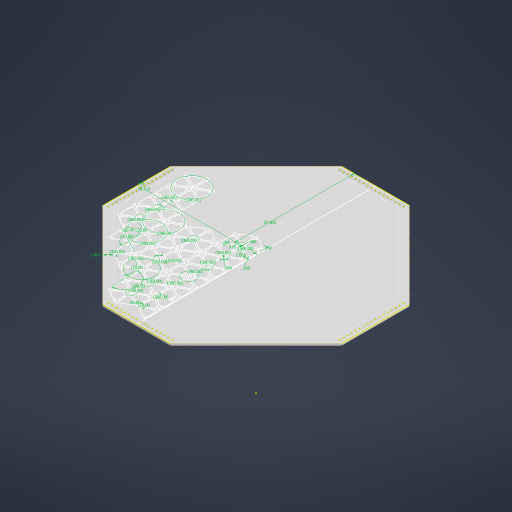
# Autodesk Inventor part: Belly Pan
Saved by Autodesk Inventor 2024.3 (Build 283343000, 343)
## iProperties
Created: 2024-11-27
Part Number: Belly Pan
Material: Generic
Document SubType Name: Modeling
Designer: kaito
Density: 1 g/cm^3
Appearance: Default
Author: kaito
Autodesk Inventor part; units mm, degrees
(part 1 of 2)
ref_plane "YZ Plane" through (0, 0, 0) normal (1, 0, 0) x (0, 1, 0)
ref_plane "XZ Plane" through (0, 0, 0) normal (0, 1, 0) x (-1, 0, 0)
ref_plane "XY Plane" through (0, 0, 0) normal (0, 0, 1) x (1, 0, 0)
sketch "Sketch1" plane through (0, 0, 0) normal (0, 1, 0) x (-1, 0, 0)
  line L0 (0, 0) -> (762, 0) construction
  line L1 (762, 0) -> (762, -762)
  line L2 (762, -762) -> (0, -762)
  line L3 (762, -273.05) -> (736.6, -273.05) construction
  line L4 (736.6, -273.05) -> (736.6, -488.95) construction
  line L5 (736.6, -488.95) -> (762, -488.95) construction
  line L6 (762, -488.95) -> (762, -273.05) construction
  line L7 (488.95, 0) -> (273.05, 0)
  line L8 (273.05, 0) -> (273.05, -25.4) construction
  line L9 (273.05, -25.4) -> (488.95, -25.4) construction
  line L10 (488.95, -25.4) -> (488.95, 0) construction
  line L11 (488.95, -762) -> (273.05, -762) construction
  line L12 (273.05, -762) -> (273.05, -736.6) construction
  line L13 (273.05, -736.6) -> (488.95, -736.6) construction
  line L14 (488.95, -736.6) -> (488.95, -762) construction
  line L15 (0, 0) -> (0, -762)
  line L16 (0, -273.05) -> (25.4, -273.05) construction
  line L17 (25.4, -273.05) -> (25.4, -488.95) construction
  line L18 (25.4, -488.95) -> (0, -488.95) construction
  line L19 (0, -488.95) -> (0, -273.05) construction
  line L20 (273.05, 0) -> (0, -273.05)
  line L21 (488.95, 0) -> (762, -273.05)
  line L22 (762, -488.95) -> (488.95, -762)
  line L23 (0, -488.95) -> (273.05, -762)
  circle A0 centre (482.6, -12.7) radius 2.4892
  circle A1 centre (469.9, -12.7) radius 2.4892
  circle A2 centre (457.2, -12.7) radius 2.4892
  circle A3 centre (444.5, -12.7) radius 2.4892
  circle A4 centre (431.8, -12.7) radius 2.4892
  circle A5 centre (419.1, -12.7) radius 2.4892
  circle A6 centre (406.4, -12.7) radius 2.4892
  circle A7 centre (393.7, -12.7) radius 2.4892
  circle A8 centre (381, -12.7) radius 2.4892
  circle A9 centre (368.3, -12.7) radius 2.4892
  circle A10 centre (355.6, -12.7) radius 2.4892
  circle A11 centre (342.9, -12.7) radius 2.4892
  circle A12 centre (330.2, -12.7) radius 2.4892
  circle A13 centre (317.5, -12.7) radius 2.4892
  circle A14 centre (304.8, -12.7) radius 2.4892
  circle A15 centre (292.1, -12.7) radius 2.4892
  circle A16 centre (279.4, -12.7) radius 2.4892
  circle A17 centre (749.3, -279.4) radius 2.4892
  circle A18 centre (749.3, -292.1) radius 2.4892
  circle A19 centre (749.3, -304.8) radius 2.4892
  circle A20 centre (749.3, -317.5) radius 2.4892
  circle A21 centre (749.3, -330.2) radius 2.4892
  circle A22 centre (749.3, -342.9) radius 2.4892
  circle A23 centre (749.3, -355.6) radius 2.4892
  circle A24 centre (749.3, -368.3) radius 2.4892
  circle A25 centre (749.3, -381) radius 2.4892
  circle A26 centre (749.3, -393.7) radius 2.4892
  circle A27 centre (749.3, -406.4) radius 2.4892
  circle A28 centre (749.3, -419.1) radius 2.4892
  circle A29 centre (749.3, -431.8) radius 2.4892
  circle A30 centre (749.3, -444.5) radius 2.4892
  circle A31 centre (749.3, -457.2) radius 2.4892
  circle A32 centre (749.3, -469.9) radius 2.4892
  circle A33 centre (749.3, -482.6) radius 2.4892
  circle A34 centre (482.6, -749.3) radius 2.4892
  circle A35 centre (469.9, -749.3) radius 2.4892
  circle A36 centre (457.2, -749.3) radius 2.4892
  circle A37 centre (444.5, -749.3) radius 2.4892
  circle A38 centre (431.8, -749.3) radius 2.4892
  circle A39 centre (419.1, -749.3) radius 2.4892
  circle A40 centre (406.4, -749.3) radius 2.4892
  circle A41 centre (393.7, -749.3) radius 2.4892
  circle A42 centre (381, -749.3) radius 2.4892
  circle A43 centre (368.3, -749.3) radius 2.4892
  circle A44 centre (355.6, -749.3) radius 2.4892
  circle A45 centre (342.9, -749.3) radius 2.4892
  circle A46 centre (330.2, -749.3) radius 2.4892
  circle A47 centre (317.5, -749.3) radius 2.4892
  circle A48 centre (304.8, -749.3) radius 2.4892
  circle A49 centre (292.1, -749.3) radius 2.4892
  circle A50 centre (279.4, -749.3) radius 2.4892
  circle A51 centre (12.7, -279.4) radius 2.4892
  circle A52 centre (12.7, -292.1) radius 2.4892
  circle A53 centre (12.7, -304.8) radius 2.4892
  circle A54 centre (12.7, -317.5) radius 2.4892
  circle A55 centre (12.7, -330.2) radius 2.4892
  circle A56 centre (12.7, -342.9) radius 2.4892
  circle A57 centre (12.7, -355.6) radius 2.4892
  circle A58 centre (12.7, -368.3) radius 2.4892
  circle A59 centre (12.7, -381) radius 2.4892
  circle A60 centre (12.7, -393.7) radius 2.4892
  circle A61 centre (12.7, -406.4) radius 2.4892
  circle A62 centre (12.7, -419.1) radius 2.4892
  circle A63 centre (12.7, -431.8) radius 2.4892
  circle A64 centre (12.7, -444.5) radius 2.4892
  circle A65 centre (12.7, -457.2) radius 2.4892
  circle A66 centre (12.7, -469.9) radius 2.4892
  circle A67 centre (12.7, -482.6) radius 2.4892
  point P0 (736.6, -381)
  point P1 (381, -25.4)
  point P2 (381, 0)
  point P3 (381, -736.6)
  point P4 (381, -762)
  point P5 (25.4, -381)
  point P6 (0, -381)
  point P7 (762, -381)
  point P8 (12.7, -273.05)
  point P9 (12.7, -488.95)
  point P10 (488.95, -12.7)
  point P11 (749.3, -273.05)
  point P12 (488.95, -749.3)
  point P13 (273.05, -762)
  point P14 (762, -488.95)
  point P15 (0, -381)
  dimension "d0" = 762
  dimension "d1" = 762
  dimension "d4" = 25.4
  dimension "d5" = 215.9
  dimension "d6" = 25.4
  dimension "d7" = 215.9
  dimension "d8" = 25.4
  dimension "d9" = 25.4
  dimension "d11" = 215.9
  dimension "d22" = 4.9784
  dimension "d23" = 6.35
  dimension "d26" = 12.7
  dimension "d31" = 4.9784
  dimension "d32" = 6.35
  dimension "d35" = 12.7
  dimension "d40" = 4.9784
  dimension "d41" = 6.35
  dimension "d44" = 12.7
  dimension "d51" = 215.9
  dimension "d60" = 4.9784
  dimension "d63" = 12.7
  constraints: 68 centre point, 48 end point, 14 midpoint, 9 parallel, 7 horizontal, 5 horizontal alignment, 5 perpendicular, 4 point on line, 4 vertical alignment, 3 vertical, 128 other
  measures "d0" distance of L1.end L2.end
  measures "d1" distance of L0.end L1.end
  measures "d4" distance of L5.end L4.end
  measures "d5" distance of L9.end L8.end
  measures "d6" distance of L8.end L7.end
  measures "d7" distance of L12.end L13.end
  measures "d8" distance of L11.end L12.end
  measures "d9" distance of L17.end L18.end
  measures "d11" distance of L3.end L4.end
  measures "d22" diameter of A0
  measures "d23" distance from line of L10 A0.centre
  measures "d26" distance of A0.centre A1.centre
  measures "d31" diameter of A17
  measures "d32" distance of point (749.3, -273.05) A17.centre
  measures "d35" distance of A17.centre A18.centre
  measures "d40" diameter of A34
  measures "d41" distance of A34.centre point (488.95, -749.3)
  measures "d44" distance of A34.centre A35.centre
  measures "d51" distance of L16.end L17.end
  measures "d60" diameter of A51
  measures "d63" distance of A51.centre A52.centre
extrude "Extrusion1" add sketch "Sketch1" along normal blind 6.35 contours L1 L22 L2 L23 L15 L20 L7 L21
sketch "Sketch4" plane through (0, 6.35, 0) normal (0, 1, 0) x (1, 0, 0)
  line L0 (-762, 488.95) -> (-762, 273.05) projected
  line L1 (0, 273.05) -> (0, 488.95) projected
  line L2 (-488.95, 0) -> (-273.05, 0) projected
  line L3 (-381, 0) -> (-381, 762)
  line L4 (-273.05, 762) -> (-488.95, 762) projected
  circle A0 centre (-428.7837, 381) radius 9.8425 construction
  line L5 (-391.0012, 361.9359) -> (-416.4013, 376.6006)
  line L6 (-416.4013, 385.3994) -> (-391.0013, 400.0641)
  line L7 (-383.3812, 395.6647) -> (-383.3812, 366.3353)
  arc A1 (-391.0012, 361.9359) -> (-383.3812, 366.3353) centre (-388.4612, 366.3353) ccw
  arc A2 (-416.4013, 385.3994) -> (-416.4013, 376.6006) centre (-413.8612, 381) ccw
  arc A3 (-383.3812, 395.6647) -> (-391.0013, 400.0641) centre (-388.4613, 395.6647) ccw
  circle A4 centre (-428.7837, 381) radius 9.8425 construction
  arc A5 (-426.4025, 393.9233) -> (-418.7825, 389.5239) centre (-421.3225, 393.9233) ccw
  line L8 (-393.3825, 404.1886) -> (-418.7825, 389.5239)
  arc A6 (-393.3825, 404.1886) -> (-393.3825, 412.9874) centre (-395.9225, 408.588) ccw
  arc A7 (-418.7825, 427.6521) -> (-426.4025, 423.2527) centre (-421.3225, 423.2527) ccw
  line L9 (-426.4025, 393.9233) -> (-426.4025, 423.2527)
  line L10 (-418.7825, 427.6521) -> (-393.3825, 412.9874)
  circle A8 centre (-428.7837, 381) radius 9.8425 construction
  arc A9 (-438.785, 389.5239) -> (-431.165, 393.9233) centre (-436.245, 393.9233) ccw
  line L11 (-431.165, 423.2527) -> (-431.165, 393.9233)
  arc A10 (-431.165, 423.2527) -> (-438.785, 427.6521) centre (-436.245, 423.2527) ccw
  arc A11 (-464.185, 412.9874) -> (-464.185, 404.1886) centre (-461.645, 408.588) ccw
  line L12 (-438.785, 389.5239) -> (-464.185, 404.1886)
  line L13 (-464.185, 412.9874) -> (-438.785, 427.6521)
  circle A12 centre (-428.7837, 381) radius 9.8425 construction
  arc A13 (-441.1662, 376.6006) -> (-441.1662, 385.3994) centre (-443.7062, 381) ccw
  line L14 (-466.5662, 400.0641) -> (-441.1662, 385.3994)
  arc A14 (-466.5662, 400.0641) -> (-474.1862, 395.6647) centre (-469.1062, 395.6647) ccw
  arc A15 (-474.1862, 366.3353) -> (-466.5662, 361.9359) centre (-469.1062, 366.3353) ccw
  line L15 (-441.1662, 376.6006) -> (-466.5662, 361.9359)
  line L16 (-474.1862, 366.3353) -> (-474.1862, 395.6647)
  circle A16 centre (-428.7837, 381) radius 9.8425 construction
  arc A17 (-431.165, 368.0767) -> (-438.785, 372.4761) centre (-436.245, 368.0767) ccw
  line L17 (-464.185, 357.8114) -> (-438.785, 372.4761)
  arc A18 (-464.185, 357.8114) -> (-464.185, 349.0126) centre (-461.645, 353.412) ccw
  arc A19 (-438.785, 334.3479) -> (-431.165, 338.7473) centre (-436.245, 338.7473) ccw
  line L18 (-431.165, 368.0767) -> (-431.165, 338.7473)
  line L19 (-438.785, 334.3479) -> (-464.185, 349.0126)
  circle A20 centre (-428.7837, 381) radius 9.8425 construction
  arc A21 (-418.7825, 372.4761) -> (-426.4025, 368.0767) centre (-421.3225, 368.0767) ccw
  line L20 (-426.4025, 338.7473) -> (-426.4025, 368.0767)
  arc A22 (-426.4025, 338.7473) -> (-418.7825, 334.3479) centre (-421.3225, 338.7473) ccw
  arc A23 (-393.3825, 349.0126) -> (-393.3825, 357.8114) centre (-395.9225, 353.412) ccw
  line L21 (-418.7825, 372.4761) -> (-393.3825, 357.8114)
  line L22 (-393.3825, 349.0126) -> (-418.7825, 334.3479)
  circle A24 centre (-428.7837, 381) radius 5.08
  circle A25 centre (-749.9958, 381) radius 6.3038 construction
  line L23 (-428.7837, 381) -> (-428.7837, 762) construction
  line L24 (-749.9958, 381) -> (-381, 381) construction
  circle A26 centre (-428.7837, 325.8241) radius 9.8425 construction
  line L25 (-441.1662, 321.4247) -> (-466.5662, 306.76)
  arc A27 (-441.1662, 321.4247) -> (-441.1662, 330.2235) centre (-443.7062, 325.8241) ccw
  line L26 (-466.5662, 344.8882) -> (-441.1662, 330.2235)
  arc A28 (-466.5662, 344.8882) -> (-474.1862, 340.4888) centre (-469.1062, 340.4888) ccw
  line L27 (-474.1862, 311.1594) -> (-474.1862, 340.4888)
  arc A29 (-474.1862, 311.1594) -> (-466.5662, 306.76) centre (-469.1062, 311.1594) ccw
  line L28 (-431.165, 312.9008) -> (-431.165, 283.5714)
  arc A30 (-431.165, 312.9008) -> (-438.785, 317.3002) centre (-436.245, 312.9008) ccw
  line L29 (-464.185, 302.6355) -> (-438.785, 317.3002)
  arc A31 (-464.185, 302.6355) -> (-464.185, 293.8367) centre (-461.645, 298.2361) ccw
  line L30 (-438.785, 279.172) -> (-464.185, 293.8367)
  arc A32 (-438.785, 279.172) -> (-431.165, 283.5714) centre (-436.245, 283.5714) ccw
  line L31 (-418.7825, 317.3002) -> (-393.3825, 302.6355)
  arc A33 (-418.7825, 317.3002) -> (-426.4025, 312.9008) centre (-421.3225, 312.9008) ccw
  line L32 (-426.4025, 283.5714) -> (-426.4025, 312.9008)
  arc A34 (-426.4025, 283.5714) -> (-418.7825, 279.172) centre (-421.3225, 283.5714) ccw
  line L33 (-393.3825, 293.8367) -> (-418.7825, 279.172)
  arc A35 (-393.3825, 293.8367) -> (-393.3825, 302.6355) centre (-395.9225, 298.2361) ccw
  line L34 (-416.4013, 330.2235) -> (-391.0012, 344.8882)
  arc A36 (-416.4013, 330.2235) -> (-416.4013, 321.4247) centre (-413.8612, 325.8241) ccw
  line L35 (-391.0012, 306.76) -> (-416.4013, 321.4247)
  arc A37 (-391.0012, 306.76) -> (-383.3812, 311.1594) centre (-388.4612, 311.1594) ccw
  line L36 (-383.3812, 340.4888) -> (-383.3812, 311.1594)
  arc A38 (-383.3812, 340.4888) -> (-391.0012, 344.8882) centre (-388.4612, 340.4888) ccw
  line L37 (-426.4025, 338.7473) -> (-426.4025, 368.0767)
  arc A39 (-426.4025, 338.7473) -> (-418.7825, 334.3479) centre (-421.3225, 338.7473) ccw
  line L38 (-393.3825, 349.0126) -> (-418.7825, 334.3479)
  arc A40 (-393.3825, 349.0126) -> (-393.3825, 357.8114) centre (-395.9225, 353.412) ccw
  line L39 (-418.7825, 372.4761) -> (-393.3825, 357.8114)
  arc A41 (-418.7825, 372.4761) -> (-426.4025, 368.0767) centre (-421.3225, 368.0767) ccw
  circle A42 centre (-428.7837, 325.8241) radius 5.08
  line L40 (-273.05, 0) -> (0, 273.05) construction
  line L41 (0, 273.05) -> (0, 488.95) construction
  line L42 (0, 488.95) -> (-273.05, 762) construction
  line L43 (-273.05, 762) -> (-488.95, 762) construction
  line L44 (-488.95, 762) -> (-762, 488.95) construction
  line L45 (-762, 488.95) -> (-762, 273.05) construction
  line L46 (-762, 273.05) -> (-488.95, 0) construction
  line L47 (-488.95, 0) -> (-273.05, 0) construction
  circle A43 centre (-12.7, 482.6) radius 2.4892 construction
  circle A44 centre (-12.7, 457.2) radius 2.4892 construction
  circle A45 centre (-12.7, 431.8) radius 2.4892 construction
  circle A46 centre (-12.7, 406.4) radius 2.4892 construction
  circle A47 centre (-12.7, 381) radius 2.4892 construction
  circle A48 centre (-12.7, 355.6) radius 2.4892 construction
  circle A49 centre (-12.7, 330.2) radius 2.4892 construction
  circle A50 centre (-12.7, 304.8) radius 2.4892 construction
  circle A51 centre (-12.7, 279.4) radius 2.4892 construction
  circle A52 centre (-292.1, 749.3) radius 2.4892 construction
  circle A53 centre (-317.5, 749.3) radius 2.4892 construction
  circle A54 centre (-342.9, 749.3) radius 2.4892 construction
  circle A55 centre (-368.3, 749.3) radius 2.4892 construction
  circle A56 centre (-393.7, 749.3) radius 2.4892 construction
  circle A57 centre (-419.1, 749.3) radius 2.4892 construction
  circle A58 centre (-444.5, 749.3) radius 2.4892 construction
  circle A59 centre (-469.9, 749.3) radius 2.4892 construction
  circle A60 centre (-749.3, 482.6) radius 2.4892 construction
  circle A61 centre (-749.3, 457.2) radius 2.4892 construction
  circle A62 centre (-749.3, 431.8) radius 2.4892 construction
  circle A63 centre (-749.3, 406.4) radius 2.4892 construction
  circle A64 centre (-749.3, 381) radius 2.4892 construction
  circle A65 centre (-749.3, 355.6) radius 2.4892 construction
  circle A66 centre (-749.3, 330.2) radius 2.4892 construction
  circle A67 centre (-749.3, 304.8) radius 2.4892 construction
  circle A68 centre (-749.3, 279.4) radius 2.4892 construction
  circle A69 centre (-292.1, 12.7) radius 2.4892 construction
  circle A70 centre (-317.5, 12.7) radius 2.4892 construction
  circle A71 centre (-342.9, 12.7) radius 2.4892 construction
  circle A72 centre (-368.3, 12.7) radius 2.4892 construction
  circle A73 centre (-393.7, 12.7) radius 2.4892 construction
  circle A74 centre (-482.6, 12.7) radius 2.4892 construction
  circle A75 centre (-469.9, 12.7) radius 2.4892 construction
  circle A76 centre (-457.2, 12.7) radius 2.4892 construction
  circle A77 centre (-444.5, 12.7) radius 2.4892 construction
  circle A78 centre (-431.8, 12.7) radius 2.4892 construction
  circle A79 centre (-419.1, 12.7) radius 2.4892 construction
  circle A80 centre (-406.4, 12.7) radius 2.4892 construction
  circle A81 centre (-381, 12.7) radius 2.4892 construction
  circle A82 centre (-355.6, 12.7) radius 2.4892 construction
  circle A83 centre (-330.2, 12.7) radius 2.4892 construction
  circle A84 centre (-304.8, 12.7) radius 2.4892 construction
  circle A85 centre (-279.4, 12.7) radius 2.4892 construction
  circle A86 centre (-749.3, 292.1) radius 2.4892 construction
  circle A87 centre (-749.3, 317.5) radius 2.4892 construction
  circle A88 centre (-749.3, 342.9) radius 2.4892 construction
  circle A89 centre (-749.3, 368.3) radius 2.4892 construction
  circle A90 centre (-749.3, 393.7) radius 2.4892 construction
  circle A91 centre (-749.3, 419.1) radius 2.4892 construction
  circle A92 centre (-749.3, 444.5) radius 2.4892 construction
  circle A93 centre (-749.3, 469.9) radius 2.4892 construction
  circle A94 centre (-482.6, 749.3) radius 2.4892 construction
  circle A95 centre (-457.2, 749.3) radius 2.4892 construction
  circle A96 centre (-431.8, 749.3) radius 2.4892 construction
  circle A97 centre (-406.4, 749.3) radius 2.4892 construction
  circle A98 centre (-381, 749.3) radius 2.4892 construction
  circle A99 centre (-355.6, 749.3) radius 2.4892 construction
  circle A100 centre (-330.2, 749.3) radius 2.4892 construction
  circle A101 centre (-304.8, 749.3) radius 2.4892 construction
  circle A102 centre (-279.4, 749.3) radius 2.4892 construction
  circle A103 centre (-12.7, 292.1) radius 2.4892 construction
  circle A104 centre (-12.7, 317.5) radius 2.4892 construction
  circle A105 centre (-12.7, 342.9) radius 2.4892 construction
  circle A106 centre (-12.7, 368.3) radius 2.4892 construction
  circle A107 centre (-12.7, 393.7) radius 2.4892 construction
  circle A108 centre (-12.7, 419.1) radius 2.4892 construction
  circle A109 centre (-12.7, 444.5) radius 2.4892 construction
  circle A110 centre (-12.7, 469.9) radius 2.4892 construction
  line L48 (-478.429, 25.4) -> (-736.6, 283.571) construction
  line L49 (-736.6, 283.571) -> (-736.6, 478.429) construction
  line L50 (-736.6, 478.429) -> (-478.429, 736.6) construction
  line L51 (-478.429, 736.6) -> (-283.571, 736.6) construction
  line L52 (-283.571, 736.6) -> (-25.4, 478.429) construction
  line L53 (-25.4, 478.429) -> (-25.4, 283.571) construction
  line L54 (-25.4, 283.571) -> (-283.571, 25.4) construction
  line L55 (-283.571, 25.4) -> (-478.429, 25.4) construction
  circle A111 centre (-428.7837, 270.6482) radius 9.8425 construction
  arc A112 (-441.1662, 266.2487) -> (-441.1662, 275.0476) centre (-443.7062, 270.6482) ccw
  line L56 (-466.5662, 289.7123) -> (-441.1662, 275.0476)
  arc A113 (-466.5662, 289.7123) -> (-474.1862, 285.3129) centre (-469.1062, 285.3129) ccw
  line L57 (-474.1862, 255.9835) -> (-474.1862, 285.3129)
  line L58 (-441.1662, 266.2487) -> (-466.5662, 251.5841)
  arc A114 (-474.1862, 255.9835) -> (-466.5662, 251.5841) centre (-469.1062, 255.9835) ccw
  arc A115 (-431.165, 257.7249) -> (-438.785, 262.1243) centre (-436.245, 257.7249) ccw
  line L59 (-464.185, 247.4596) -> (-438.785, 262.1243)
  arc A116 (-464.185, 247.4596) -> (-464.185, 238.6608) centre (-461.645, 243.0602) ccw
  line L60 (-438.785, 223.9961) -> (-464.185, 238.6608)
  line L61 (-431.165, 257.7249) -> (-431.165, 228.3955)
  arc A117 (-438.785, 223.9961) -> (-431.165, 228.3955) centre (-436.245, 228.3955) ccw
  arc A118 (-418.7825, 262.1243) -> (-426.4025, 257.7249) centre (-421.3225, 257.7249) ccw
  line L62 (-426.4025, 228.3955) -> (-426.4025, 257.7249)
  arc A119 (-426.4025, 228.3955) -> (-418.7825, 223.9961) centre (-421.3225, 228.3955) ccw
  line L63 (-393.3825, 238.6608) -> (-418.7825, 223.9961)
  line L64 (-418.7825, 262.1243) -> (-393.3825, 247.4596)
  arc A120 (-393.3825, 238.6608) -> (-393.3825, 247.4596) centre (-395.9225, 243.0602) ccw
  arc A121 (-416.4012, 275.0476) -> (-416.4012, 266.2487) centre (-413.8612, 270.6482) ccw
  line L65 (-391.0012, 251.5841) -> (-416.4012, 266.2487)
  arc A122 (-391.0012, 251.5841) -> (-383.3812, 255.9835) centre (-388.4612, 255.9835) ccw
  line L66 (-383.3812, 285.3129) -> (-383.3812, 255.9835)
  line L67 (-416.4012, 275.0476) -> (-391.0012, 289.7123)
  arc A123 (-383.3812, 285.3129) -> (-391.0012, 289.7123) centre (-388.4612, 285.3129) ccw
  arc A124 (-426.4025, 283.5714) -> (-418.7825, 279.172) centre (-421.3225, 283.5714) ccw
  line L68 (-393.3825, 293.8367) -> (-418.7825, 279.172)
  arc A125 (-393.3825, 293.8367) -> (-393.3825, 302.6355) centre (-395.9225, 298.2361) ccw
  line L69 (-418.7825, 317.3002) -> (-393.3825, 302.6355)
  line L70 (-426.4025, 283.5714) -> (-426.4025, 312.9008)
  arc A126 (-418.7825, 317.3002) -> (-426.4025, 312.9008) centre (-421.3225, 312.9008) ccw
  circle A127 centre (-428.7837, 215.4722) radius 9.8425 construction
  line L71 (-466.5662, 234.5363) -> (-441.1662, 219.8716)
  arc A128 (-441.1663, 211.0728) -> (-441.1662, 219.8716) centre (-443.7062, 215.4722) ccw
  line L72 (-441.1663, 211.0728) -> (-466.5663, 196.4081)
  arc A129 (-474.1862, 200.8075) -> (-466.5663, 196.4081) centre (-469.1062, 200.8075) ccw
  line L73 (-474.1862, 200.8075) -> (-474.1862, 230.1369)
  arc A130 (-466.5662, 234.5363) -> (-474.1862, 230.1369) centre (-469.1062, 230.1369) ccw
  line L74 (-464.185, 192.2837) -> (-438.785, 206.9484)
  arc A131 (-431.165, 202.549) -> (-438.785, 206.9484) centre (-436.245, 202.549) ccw
  line L75 (-431.165, 202.549) -> (-431.165, 173.2196)
  arc A132 (-438.785, 168.8202) -> (-431.165, 173.2196) centre (-436.245, 173.2196) ccw
  line L76 (-438.785, 168.8202) -> (-464.185, 183.4849)
  arc A133 (-464.185, 192.2837) -> (-464.185, 183.4849) centre (-461.645, 187.8843) ccw
  line L77 (-426.4025, 173.2196) -> (-426.4025, 202.549)
  arc A134 (-418.7825, 206.9484) -> (-426.4025, 202.549) centre (-421.3225, 202.549) ccw
  line L78 (-418.7825, 206.9484) -> (-393.3825, 192.2837)
  arc A135 (-393.3825, 183.4849) -> (-393.3825, 192.2837) centre (-395.9225, 187.8843) ccw
  line L79 (-393.3825, 183.4849) -> (-418.7825, 168.8202)
  arc A136 (-426.4025, 173.2196) -> (-418.7825, 168.8202) centre (-421.3225, 173.2196) ccw
  line L80 (-391.0012, 196.4081) -> (-416.4012, 211.0728)
  arc A137 (-416.4012, 219.8716) -> (-416.4012, 211.0728) centre (-413.8612, 215.4722) ccw
  line L81 (-416.4012, 219.8716) -> (-391.0012, 234.5363)
  arc A138 (-383.3812, 230.1369) -> (-391.0012, 234.5363) centre (-388.4612, 230.1369) ccw
  line L82 (-383.3812, 230.1369) -> (-383.3812, 200.8075)
  arc A139 (-391.0012, 196.4081) -> (-383.3812, 200.8075) centre (-388.4612, 200.8075) ccw
  line L83 (-393.3825, 238.6608) -> (-418.7825, 223.9961)
  arc A140 (-426.4025, 228.3955) -> (-418.7825, 223.9961) centre (-421.3225, 228.3955) ccw
  line L84 (-426.4025, 228.3955) -> (-426.4025, 257.7249)
  arc A141 (-418.7825, 262.1243) -> (-426.4025, 257.7249) centre (-421.3225, 257.7249) ccw
  line L85 (-418.7825, 262.1243) -> (-393.3825, 247.4596)
  arc A142 (-393.3825, 238.6608) -> (-393.3825, 247.4596) centre (-395.9225, 243.0602) ccw
  circle A143 centre (-428.7837, 160.2963) radius 9.8425 construction
  line L86 (-441.1662, 155.8969) -> (-466.5662, 141.2322)
  arc A144 (-441.1662, 155.8969) -> (-441.1662, 164.6957) centre (-443.7062, 160.2963) ccw
  line L87 (-466.5662, 179.3604) -> (-441.1662, 164.6957)
  arc A145 (-466.5662, 179.3604) -> (-474.1862, 174.961) centre (-469.1062, 174.961) ccw
  line L88 (-474.1862, 145.6316) -> (-474.1862, 174.961)
  arc A146 (-474.1862, 145.6316) -> (-466.5662, 141.2322) centre (-469.1062, 145.6316) ccw
  line L89 (-431.165, 147.373) -> (-431.165, 118.0437)
  arc A147 (-431.165, 147.373) -> (-438.785, 151.7725) centre (-436.245, 147.373) ccw
  line L90 (-464.185, 137.1078) -> (-438.785, 151.7725)
  arc A148 (-464.185, 137.1078) -> (-464.185, 128.3089) centre (-461.645, 132.7084) ccw
  line L91 (-438.785, 113.6442) -> (-464.185, 128.3089)
  arc A149 (-438.785, 113.6442) -> (-431.165, 118.0437) centre (-436.245, 118.0437) ccw
  line L92 (-418.7825, 151.7725) -> (-393.3825, 137.1078)
  arc A150 (-418.7825, 151.7725) -> (-426.4025, 147.373) centre (-421.3225, 147.373) ccw
  line L93 (-426.4025, 118.0437) -> (-426.4025, 147.373)
  arc A151 (-426.4025, 118.0437) -> (-418.7825, 113.6442) centre (-421.3225, 118.0437) ccw
  line L94 (-393.3825, 128.3089) -> (-418.7825, 113.6442)
  arc A152 (-393.3825, 128.3089) -> (-393.3825, 137.1078) centre (-395.9225, 132.7084) ccw
  line L95 (-416.4012, 164.6957) -> (-391.0012, 179.3604)
  arc A153 (-416.4012, 164.6957) -> (-416.4012, 155.8969) centre (-413.8612, 160.2963) ccw
  line L96 (-391.0012, 141.2322) -> (-416.4012, 155.8969)
  arc A154 (-391.0012, 141.2322) -> (-383.3812, 145.6316) centre (-388.4612, 145.6316) ccw
  line L97 (-383.3812, 174.961) -> (-383.3812, 145.6316)
  arc A155 (-383.3812, 174.961) -> (-391.0012, 179.3604) centre (-388.4612, 174.961) ccw
  line L98 (-426.4025, 173.2196) -> (-426.4025, 202.549)
  arc A156 (-426.4025, 173.2196) -> (-418.7825, 168.8202) centre (-421.3225, 173.2196) ccw
  line L99 (-393.3825, 183.4849) -> (-418.7825, 168.8202)
  arc A157 (-393.3825, 183.4849) -> (-393.3825, 192.2837) centre (-395.9225, 187.8843) ccw
  line L100 (-418.7825, 206.9484) -> (-393.3825, 192.2837)
  arc A158 (-418.7825, 206.9484) -> (-426.4025, 202.549) centre (-421.3225, 202.549) ccw
  circle A159 centre (-428.7837, 105.1204) radius 9.8425 construction
  arc A160 (-438.785, 113.6442) -> (-431.165, 118.0437) centre (-436.245, 118.0437) ccw
  line L101 (-431.165, 147.373) -> (-431.165, 118.0437)
  arc A161 (-431.165, 147.373) -> (-438.785, 151.7725) centre (-436.245, 147.373) ccw
  line L102 (-464.185, 137.1078) -> (-438.785, 151.7725)
  line L103 (-438.785, 113.6442) -> (-464.185, 128.3089)
  arc A162 (-464.185, 137.1078) -> (-464.185, 128.3089) centre (-461.645, 132.7084) ccw
  arc A163 (-441.1662, 100.721) -> (-441.1662, 109.5198) centre (-443.7062, 105.1204) ccw
  line L104 (-466.5662, 124.1845) -> (-441.1662, 109.5198)
  arc A164 (-466.5662, 124.1845) -> (-474.1862, 119.7851) centre (-469.1062, 119.7851) ccw
  line L105 (-474.1862, 90.4557) -> (-474.1862, 119.7851)
  line L106 (-441.1662, 100.721) -> (-466.5662, 86.0563)
  arc A165 (-474.1862, 90.4557) -> (-466.5662, 86.0563) centre (-469.1062, 90.4557) ccw
  arc A166 (-431.165, 92.1971) -> (-438.785, 96.5965) centre (-436.245, 92.1971) ccw
  line L107 (-464.185, 81.9318) -> (-438.785, 96.5965)
  arc A167 (-464.185, 81.9318) -> (-464.185, 73.133) centre (-461.645, 77.5324) ccw
  line L108 (-438.785, 58.4683) -> (-464.185, 73.133)
  line L109 (-431.165, 92.1971) -> (-431.165, 62.8677)
  arc A168 (-438.785, 58.4683) -> (-431.165, 62.8677) centre (-436.245, 62.8677) ccw
  arc A169 (-418.7825, 96.5965) -> (-426.4025, 92.1971) centre (-421.3225, 92.1971) ccw
  line L110 (-426.4025, 62.8677) -> (-426.4025, 92.1971)
  arc A170 (-426.4025, 62.8677) -> (-418.7825, 58.4683) centre (-421.3225, 62.8677) ccw
  line L111 (-393.3825, 73.133) -> (-418.7825, 58.4683)
  line L112 (-418.7825, 96.5965) -> (-393.3825, 81.9318)
  arc A171 (-393.3825, 73.133) -> (-393.3825, 81.9318) centre (-395.9225, 77.5324) ccw
  arc A172 (-416.4012, 109.5198) -> (-416.4012, 100.721) centre (-413.8612, 105.1204) ccw
  line L113 (-391.0012, 86.0563) -> (-416.4012, 100.721)
  arc A173 (-391.0012, 86.0563) -> (-383.3812, 90.4557) centre (-388.4612, 90.4557) ccw
  line L114 (-383.3812, 119.7851) -> (-383.3812, 90.4557)
  line L115 (-416.4012, 109.5198) -> (-391.0012, 124.1845)
  arc A174 (-383.3812, 119.7851) -> (-391.0012, 124.1845) centre (-388.4612, 119.7851) ccw
  circle A175 centre (-428.7837, 49.9445) radius 9.8425 construction
  arc A176 (-416.4012, 54.3439) -> (-416.4012, 45.5451) centre (-413.8612, 49.9445) ccw
  line L116 (-416.4012, 54.3439) -> (-391.0012, 69.0086)
  arc A177 (-383.3812, 64.6092) -> (-391.0012, 69.0086) centre (-388.4612, 64.6092) ccw
  line L117 (-383.3812, 64.6092) -> (-383.3812, 35.2798)
  arc A178 (-391.0012, 30.8804) -> (-383.3812, 35.2798) centre (-388.4612, 35.2798) ccw
  line L118 (-391.0012, 30.8804) -> (-416.4012, 45.5451)
  arc A179 (-441.1662, 45.5451) -> (-441.1662, 54.3439) centre (-443.7062, 49.9445) ccw
  line L119 (-441.1662, 45.5451) -> (-466.5662, 30.8804)
  arc A180 (-474.1862, 35.2798) -> (-466.5662, 30.8804) centre (-469.1062, 35.2798) ccw
  line L120 (-474.1862, 35.2798) -> (-474.1862, 64.6092)
  arc A181 (-466.5662, 69.0086) -> (-474.1862, 64.6092) centre (-469.1062, 64.6092) ccw
  line L121 (-466.5662, 69.0086) -> (-441.1662, 54.3439)
  circle A182 centre (-476.5675, 77.5324) radius 9.8425 construction
  line L122 (-486.5687, 86.0563) -> (-511.9687, 100.721)
  arc A183 (-486.5687, 86.0563) -> (-478.9487, 90.4557) centre (-484.0287, 90.4557) ccw
  line L123 (-478.9487, 119.7851) -> (-478.9487, 90.4557)
  arc A184 (-478.9487, 119.7851) -> (-486.5687, 124.1845) centre (-484.0287, 119.7851) ccw
  arc A185 (-511.9687, 109.5198) -> (-511.9687, 100.721) centre (-509.4287, 105.1204) ccw
  line L124 (-511.9687, 109.5198) -> (-486.5687, 124.1845)
  line L125 (-488.95, 73.133) -> (-514.35, 58.4683)
  arc A186 (-488.95, 73.133) -> (-488.95, 81.9318) centre (-491.49, 77.5324) ccw
  line L126 (-514.35, 96.5965) -> (-488.95, 81.9318)
  arc A187 (-514.35, 96.5965) -> (-521.97, 92.1971) centre (-516.89, 92.1971) ccw
  arc A188 (-521.97, 62.8677) -> (-514.35, 58.4683) centre (-516.89, 62.8677) ccw
  line L127 (-521.97, 62.8677) -> (-521.97, 92.1971)
  line L128 (-478.9487, 64.6092) -> (-478.9487, 35.2798)
  arc A189 (-478.9487, 64.6092) -> (-486.5687, 69.0086) centre (-484.0287, 64.6092) ccw
  line L129 (-511.9687, 54.3439) -> (-486.5687, 69.0086)
  arc A190 (-511.9687, 54.3439) -> (-511.9687, 45.5451) centre (-509.4287, 49.9445) ccw
  arc A191 (-486.5687, 30.8804) -> (-478.9487, 35.2798) centre (-484.0287, 35.2798) ccw
  line L130 (-486.5687, 30.8804) -> (-511.9687, 45.5451)
  line L131 (-466.5662, 69.0086) -> (-441.1662, 54.3439)
  arc A192 (-466.5662, 69.0086) -> (-474.1862, 64.6092) centre (-469.1062, 64.6092) ccw
  line L132 (-474.1862, 35.2798) -> (-474.1862, 64.6092)
  arc A193 (-474.1862, 35.2798) -> (-466.5662, 30.8804) centre (-469.1062, 35.2798) ccw
  arc A194 (-441.1662, 45.5451) -> (-441.1662, 54.3439) centre (-443.7062, 49.9445) ccw
  line L133 (-441.1662, 45.5451) -> (-466.5662, 30.8804)
  line L134 (-464.185, 81.9318) -> (-438.785, 96.5965)
  arc A195 (-464.185, 81.9318) -> (-464.185, 73.133) centre (-461.645, 77.5324) ccw
  line L135 (-438.785, 58.4683) -> (-464.185, 73.133)
  arc A196 (-438.785, 58.4683) -> (-431.165, 62.8677) centre (-436.245, 62.8677) ccw
  arc A197 (-431.165, 92.1971) -> (-438.785, 96.5965) centre (-436.245, 92.1971) ccw
  line L136 (-431.165, 92.1971) -> (-431.165, 62.8677)
  circle A198 centre (-476.5675, 132.7084) radius 9.8425 construction
  arc A199 (-486.5687, 141.2322) -> (-478.9487, 145.6316) centre (-484.0287, 145.6316) ccw
  line L137 (-486.5687, 141.2322) -> (-511.9687, 155.8969)
  arc A200 (-511.9687, 164.6957) -> (-511.9687, 155.8969) centre (-509.4287, 160.2963) ccw
  line L138 (-511.9687, 164.6957) -> (-486.5687, 179.3604)
  circle A201 centre (-476.5675, 187.8843) radius 9.8425 construction
  line L139 (-478.9487, 174.961) -> (-478.9487, 145.6316)
  arc A202 (-478.9487, 174.961) -> (-486.5687, 179.3604) centre (-484.0287, 174.961) ccw
  arc A203 (-488.95, 128.3089) -> (-488.95, 137.1078) centre (-491.49, 132.7084) ccw
  line L140 (-488.95, 128.3089) -> (-514.35, 113.6442)
  arc A204 (-521.97, 118.0437) -> (-514.35, 113.6442) centre (-516.89, 118.0437) ccw
  line L141 (-521.97, 118.0437) -> (-521.97, 147.373)
  circle A205 centre (-524.3512, 160.2963) radius 9.8425 construction
  line L142 (-514.35, 151.7725) -> (-488.95, 137.1078)
  arc A206 (-514.35, 151.7725) -> (-521.97, 147.373) centre (-516.89, 147.373) ccw
  arc A207 (-478.9487, 119.7851) -> (-486.5687, 124.1845) centre (-484.0287, 119.7851) ccw
  line L143 (-478.9487, 119.7851) -> (-478.9487, 90.4557)
  arc A208 (-486.5687, 86.0563) -> (-478.9487, 90.4557) centre (-484.0287, 90.4557) ccw
  line L144 (-486.5687, 86.0563) -> (-511.9687, 100.721)
  circle A209 centre (-524.3512, 105.1204) radius 9.8425 construction
  line L145 (-511.9687, 109.5198) -> (-486.5687, 124.1845)
  arc A210 (-511.9687, 109.5198) -> (-511.9687, 100.721) centre (-509.4287, 105.1204) ccw
  arc A211 (-466.5662, 124.1845) -> (-474.1862, 119.7851) centre (-469.1062, 119.7851) ccw
  line L146 (-466.5662, 124.1845) -> (-441.1662, 109.5198)
  arc A212 (-441.1662, 100.721) -> (-441.1662, 109.5198) centre (-443.7062, 105.1204) ccw
  line L147 (-441.1662, 100.721) -> (-466.5662, 86.0563)
  circle A213 centre (-476.5675, 77.5324) radius 9.8425 construction
  line L148 (-474.1862, 90.4557) -> (-474.1862, 119.7851)
  arc A214 (-474.1862, 90.4557) -> (-466.5662, 86.0563) centre (-469.1062, 90.4557) ccw
  arc A215 (-464.185, 137.1078) -> (-464.185, 128.3089) centre (-461.645, 132.7084) ccw
  line L149 (-464.185, 137.1078) -> (-438.785, 151.7725)
  arc A216 (-431.165, 147.373) -> (-438.785, 151.7725) centre (-436.245, 147.373) ccw
  line L150 (-431.165, 147.373) -> (-431.165, 118.0437)
  circle A217 centre (-428.7837, 105.1204) radius 9.8425 construction
  line L151 (-438.785, 113.6442) -> (-464.185, 128.3089)
  arc A218 (-438.785, 113.6442) -> (-431.165, 118.0437) centre (-436.245, 118.0437) ccw
  line L152 (-486.5687, 86.0563) -> (-511.9687, 100.721)
  arc A219 (-486.5687, 86.0563) -> (-478.9487, 90.4557) centre (-484.0287, 90.4557) ccw
  line L153 (-478.9487, 119.7851) -> (-478.9487, 90.4557)
  arc A220 (-478.9487, 119.7851) -> (-486.5687, 124.1845) centre (-484.0287, 119.7851) ccw
  line L154 (-511.9687, 109.5198) -> (-486.5687, 124.1845)
  arc A221 (-511.9687, 109.5198) -> (-511.9687, 100.721) centre (-509.4287, 105.1204) ccw
  line L155 (-488.95, 128.3089) -> (-514.35, 113.6442)
  arc A222 (-488.95, 128.3089) -> (-488.95, 137.1078) centre (-491.49, 132.7084) ccw
  line L156 (-514.35, 151.7725) -> (-488.95, 137.1078)
  arc A223 (-514.35, 151.7725) -> (-521.97, 147.373) centre (-516.89, 147.373) ccw
  line L157 (-521.97, 118.0437) -> (-521.97, 147.373)
  arc A224 (-521.97, 118.0437) -> (-514.35, 113.6442) centre (-516.89, 118.0437) ccw
  line L158 (-526.7325, 147.373) -> (-526.7325, 118.0437)
  arc A225 (-526.7325, 147.373) -> (-534.3525, 151.7725) centre (-531.8125, 147.373) ccw
  line L159 (-559.7525, 137.1078) -> (-534.3525, 151.7725)
  arc A226 (-559.7525, 137.1078) -> (-559.7525, 128.3089) centre (-557.2125, 132.7084) ccw
  line L160 (-534.3525, 113.6442) -> (-559.7525, 128.3089)
  arc A227 (-534.3525, 113.6442) -> (-526.7325, 118.0437) centre (-531.8125, 118.0437) ccw
  circle A228 centre (-572.135, 132.7084) radius 9.8425 construction
  line L161 (-536.7337, 155.8969) -> (-562.1337, 141.2322)
  arc A229 (-536.7337, 155.8969) -> (-536.7337, 164.6957) centre (-539.2737, 160.2963) ccw
  line L162 (-562.1337, 179.3604) -> (-536.7337, 164.6957)
  arc A230 (-562.1337, 179.3604) -> (-569.7537, 174.961) centre (-564.6737, 174.961) ccw
  line L163 (-569.7537, 145.6316) -> (-569.7537, 174.961)
  arc A231 (-569.7537, 145.6316) -> (-562.1337, 141.2322) centre (-564.6737, 145.6316) ccw
  line L164 (-574.5162, 174.961) -> (-574.5162, 145.6316)
  arc A232 (-574.5162, 174.961) -> (-582.1362, 179.3604) centre (-579.5962, 174.961) ccw
  line L165 (-607.5362, 164.6957) -> (-582.1362, 179.3604)
  arc A233 (-607.5362, 164.6957) -> (-607.5362, 155.8969) centre (-604.9962, 160.2963) ccw
  line L166 (-582.1362, 141.2322) -> (-607.5362, 155.8969)
  arc A234 (-582.1362, 141.2322) -> (-574.5162, 145.6316) centre (-579.5962, 145.6316) ccw
  line L167 (-559.7525, 137.1078) -> (-534.3525, 151.7725)
  arc A235 (-526.7325, 147.373) -> (-534.3525, 151.7725) centre (-531.8125, 147.373) ccw
  line L168 (-526.7325, 147.373) -> (-526.7325, 118.0437)
  arc A236 (-534.3525, 113.6442) -> (-526.7325, 118.0437) centre (-531.8125, 118.0437) ccw
  line L169 (-534.3525, 113.6442) -> (-559.7525, 128.3089)
  arc A237 (-559.7525, 137.1078) -> (-559.7525, 128.3089) centre (-557.2125, 132.7084) ccw
  line L170 (-521.97, 118.0437) -> (-521.97, 147.373)
  arc A238 (-514.35, 151.7725) -> (-521.97, 147.373) centre (-516.89, 147.373) ccw
  line L171 (-514.35, 151.7725) -> (-488.95, 137.1078)
  arc A239 (-488.95, 128.3089) -> (-488.95, 137.1078) centre (-491.49, 132.7084) ccw
  line L172 (-488.95, 128.3089) -> (-514.35, 113.6442)
  arc A240 (-521.97, 118.0437) -> (-514.35, 113.6442) centre (-516.89, 118.0437) ccw
  line L173 (-486.5687, 141.2322) -> (-511.9687, 155.8969)
  arc A241 (-511.9687, 164.6957) -> (-511.9687, 155.8969) centre (-509.4287, 160.2963) ccw
  line L174 (-511.9687, 164.6957) -> (-486.5687, 179.3604)
  arc A242 (-478.9487, 174.961) -> (-486.5687, 179.3604) centre (-484.0287, 174.961) ccw
  line L175 (-478.9487, 174.961) -> (-478.9487, 145.6316)
  arc A243 (-486.5687, 141.2322) -> (-478.9487, 145.6316) centre (-484.0287, 145.6316) ccw
  line L176 (-488.95, 183.4849) -> (-514.35, 168.8202)
  arc A244 (-521.97, 173.2196) -> (-514.35, 168.8202) centre (-516.89, 173.2196) ccw
  line L177 (-521.97, 173.2196) -> (-521.97, 202.549)
  arc A245 (-514.35, 206.9484) -> (-521.97, 202.549) centre (-516.89, 202.549) ccw
  line L178 (-514.35, 206.9484) -> (-488.95, 192.2837)
  arc A246 (-488.95, 183.4849) -> (-488.95, 192.2837) centre (-491.49, 187.8843) ccw
  line L179 (-526.7325, 202.549) -> (-526.7325, 173.2196)
  arc A247 (-534.3525, 168.8202) -> (-526.7325, 173.2196) centre (-531.8125, 173.2196) ccw
  line L180 (-534.3525, 168.8202) -> (-559.7525, 183.4849)
  arc A248 (-559.7525, 192.2837) -> (-559.7525, 183.4849) centre (-557.2125, 187.8843) ccw
  line L181 (-559.7525, 192.2837) -> (-534.3525, 206.9484)
  arc A249 (-526.7325, 202.549) -> (-534.3525, 206.9484) centre (-531.8125, 202.549) ccw
  circle A250 centre (-572.135, 187.8843) radius 9.8425 construction
  arc A251 (-569.7538, 145.6316) -> (-562.1338, 141.2322) centre (-564.6738, 145.6316) ccw
  line L182 (-536.7337, 155.8969) -> (-562.1338, 141.2322)
  arc A252 (-536.7337, 155.8969) -> (-536.7338, 164.6957) centre (-539.2738, 160.2963) ccw
  line L183 (-562.1337, 179.3604) -> (-536.7338, 164.6957)
  line L184 (-569.7538, 145.6316) -> (-569.7538, 174.961)
  arc A253 (-562.1337, 179.3604) -> (-569.7538, 174.961) centre (-564.6738, 174.961) ccw
  arc A254 (-534.3525, 168.8202) -> (-526.7325, 173.2196) centre (-531.8125, 173.2196) ccw
  line L185 (-526.7325, 202.549) -> (-526.7325, 173.2196)
  arc A255 (-526.7325, 202.549) -> (-534.3525, 206.9484) centre (-531.8125, 202.549) ccw
  line L186 (-559.7525, 192.2837) -> (-534.3525, 206.9484)
  line L187 (-534.3525, 168.8202) -> (-559.7525, 183.4849)
  arc A256 (-559.7525, 192.2837) -> (-559.7525, 183.4849) centre (-557.2125, 187.8843) ccw
  arc A257 (-536.7337, 211.0728) -> (-536.7337, 219.8716) centre (-539.2737, 215.4722) ccw
  line L188 (-562.1337, 234.5363) -> (-536.7337, 219.8716)
  arc A258 (-562.1337, 234.5363) -> (-569.7537, 230.1369) centre (-564.6737, 230.1369) ccw
  line L189 (-569.7537, 200.8075) -> (-569.7537, 230.1369)
  line L190 (-536.7337, 211.0728) -> (-562.1337, 196.4081)
  arc A259 (-569.7537, 200.8075) -> (-562.1337, 196.4081) centre (-564.6737, 200.8075) ccw
  arc A260 (-574.5162, 230.1369) -> (-582.1362, 234.5363) centre (-579.5962, 230.1369) ccw
  line L191 (-607.5362, 219.8716) -> (-582.1362, 234.5363)
  arc A261 (-607.5362, 219.8716) -> (-607.5362, 211.0728) centre (-604.9962, 215.4722) ccw
  line L192 (-582.1362, 196.4081) -> (-607.5362, 211.0728)
  line L193 (-574.5162, 230.1369) -> (-574.5162, 200.8075)
  arc A262 (-582.1362, 196.4081) -> (-574.5162, 200.8075) centre (-579.5962, 200.8075) ccw
  arc A263 (-609.9175, 206.9484) -> (-617.5375, 202.549) centre (-612.4575, 202.549) ccw
  line L194 (-617.5375, 173.2196) -> (-617.5375, 202.549)
  arc A264 (-617.5375, 173.2196) -> (-609.9175, 168.8202) centre (-612.4575, 173.2196) ccw
  line L195 (-584.5175, 183.4849) -> (-609.9175, 168.8202)
  line L196 (-609.9175, 206.9484) -> (-584.5175, 192.2837)
  arc A265 (-584.5175, 183.4849) -> (-584.5175, 192.2837) centre (-587.0575, 187.8843) ccw
  circle A266 centre (-619.9187, 215.4722) radius 9.8425 construction
  line L197 (-584.5175, 238.6608) -> (-609.9175, 223.9961)
  arc A267 (-584.5175, 238.6608) -> (-584.5175, 247.4596) centre (-587.0575, 243.0602) ccw
  line L198 (-609.9175, 262.1243) -> (-584.5175, 247.4596)
  arc A268 (-609.9175, 262.1243) -> (-617.5375, 257.7249) centre (-612.4575, 257.7249) ccw
  line L199 (-617.5375, 228.3955) -> (-617.5375, 257.7249)
  arc A269 (-617.5375, 228.3955) -> (-609.9175, 223.9961) centre (-612.4575, 228.3955) ccw
  line L200 (-622.3, 257.7249) -> (-622.3, 228.3955)
  arc A270 (-622.3, 257.7249) -> (-629.92, 262.1243) centre (-627.38, 257.7249) ccw
  line L201 (-655.32, 247.4596) -> (-629.92, 262.1243)
  arc A271 (-655.32, 247.4596) -> (-655.32, 238.6608) centre (-652.78, 243.0602) ccw
  line L202 (-629.92, 223.9961) -> (-655.32, 238.6608)
  arc A272 (-629.92, 223.9961) -> (-622.3, 228.3955) centre (-627.38, 228.3955) ccw
  circle A273 centre (-667.7025, 243.0602) radius 9.8425 construction
  line L203 (-632.3012, 266.2487) -> (-657.7013, 251.5841)
  arc A274 (-632.3012, 266.2487) -> (-632.3013, 275.0476) centre (-634.8413, 270.6482) ccw
  line L204 (-657.7012, 289.7123) -> (-632.3013, 275.0476)
  arc A275 (-657.7012, 289.7123) -> (-665.3213, 285.3129) centre (-660.2413, 285.3129) ccw
  line L205 (-665.3213, 255.9835) -> (-665.3213, 285.3129)
  arc A276 (-665.3213, 255.9835) -> (-657.7013, 251.5841) centre (-660.2413, 255.9835) ccw
  line L206 (-670.0837, 285.3129) -> (-670.0838, 255.9835)
  arc A277 (-670.0837, 285.3129) -> (-677.7037, 289.7123) centre (-675.1637, 285.3129) ccw
  line L207 (-703.1037, 275.0476) -> (-677.7037, 289.7123)
  arc A278 (-703.1037, 275.0476) -> (-703.1037, 266.2487) centre (-700.5638, 270.6482) ccw
  line L208 (-677.7038, 251.5841) -> (-703.1037, 266.2487)
  arc A279 (-677.7038, 251.5841) -> (-670.0838, 255.9835) centre (-675.1637, 255.9835) ccw
  line L209 (-657.7012, 234.5363) -> (-632.3012, 219.8716)
  arc A280 (-657.7012, 234.5363) -> (-665.3212, 230.1369) centre (-660.2412, 230.1369) ccw
  line L210 (-665.3212, 200.8075) -> (-665.3212, 230.1369)
  arc A281 (-665.3212, 200.8075) -> (-657.7012, 196.4081) centre (-660.2412, 200.8075) ccw
  line L211 (-632.3012, 211.0728) -> (-657.7012, 196.4081)
  arc A282 (-632.3012, 211.0728) -> (-632.3012, 219.8716) centre (-634.8412, 215.4722) ccw
  circle A283 centre (-667.7025, 298.2361) radius 9.8425 construction
  line L212 (-657.7012, 289.7123) -> (-632.3012, 275.0476)
  arc A284 (-632.3012, 266.2487) -> (-632.3012, 275.0476) centre (-634.8412, 270.6482) ccw
  line L213 (-632.3012, 266.2487) -> (-657.7012, 251.5841)
  arc A285 (-665.3212, 255.9835) -> (-657.7012, 251.5841) centre (-660.2412, 255.9835) ccw
  line L214 (-665.3212, 255.9835) -> (-665.3212, 285.3129)
  arc A286 (-657.7012, 289.7123) -> (-665.3212, 285.3129) centre (-660.2412, 285.3129) ccw
  line L215 (-655.32, 302.6355) -> (-629.92, 317.3002)
  arc A287 (-622.3, 312.9008) -> (-629.92, 317.3002) centre (-627.38, 312.9008) ccw
  line L216 (-622.3, 312.9008) -> (-622.3, 283.5714)
  arc A288 (-629.92, 279.172) -> (-622.3, 283.5714) centre (-627.38, 283.5714) ccw
  line L217 (-629.92, 279.172) -> (-655.32, 293.8367)
  arc A289 (-655.32, 302.6355) -> (-655.32, 293.8367) centre (-652.78, 298.2361) ccw
  line L218 (-665.3212, 311.1594) -> (-665.3212, 340.4888)
  arc A290 (-657.7012, 344.8882) -> (-665.3212, 340.4888) centre (-660.2412, 340.4888) ccw
  line L219 (-657.7012, 344.8882) -> (-632.3012, 330.2235)
  arc A291 (-632.3012, 321.4247) -> (-632.3012, 330.2235) centre (-634.8412, 325.8241) ccw
  line L220 (-632.3012, 321.4247) -> (-657.7012, 306.76)
  arc A292 (-665.3212, 311.1594) -> (-657.7012, 306.76) centre (-660.2412, 311.1594) ccw
  line L221 (-677.7038, 306.76) -> (-703.1038, 321.4247)
  arc A293 (-703.1038, 330.2235) -> (-703.1038, 321.4247) centre (-700.5638, 325.8241) ccw
  line L222 (-703.1038, 330.2235) -> (-677.7038, 344.8882)
  arc A294 (-670.0838, 340.4888) -> (-677.7038, 344.8882) centre (-675.1638, 340.4888) ccw
  line L223 (-670.0838, 340.4888) -> (-670.0838, 311.1594)
  arc A295 (-677.7038, 306.76) -> (-670.0838, 311.1594) centre (-675.1638, 311.1594) ccw
  line L224 (-680.085, 293.8367) -> (-705.485, 279.172)
  arc A296 (-713.105, 283.5714) -> (-705.485, 279.172) centre (-708.025, 283.5714) ccw
  line L225 (-713.105, 283.5714) -> (-713.105, 312.9008)
  arc A297 (-705.485, 317.3002) -> (-713.105, 312.9008) centre (-708.025, 312.9008) ccw
  line L226 (-705.485, 317.3002) -> (-680.085, 302.6355)
  arc A298 (-680.085, 293.8367) -> (-680.085, 302.6355) centre (-682.625, 298.2361) ccw
  circle A299 centre (-667.7025, 353.412) radius 9.8425 construction
  line L227 (-657.7013, 344.8882) -> (-632.3013, 330.2235)
  arc A300 (-632.3013, 321.4247) -> (-632.3013, 330.2235) centre (-634.8413, 325.8241) ccw
  line L228 (-632.3013, 321.4247) -> (-657.7013, 306.76)
  arc A301 (-665.3213, 311.1594) -> (-657.7013, 306.76) centre (-660.2413, 311.1594) ccw
  line L229 (-665.3213, 311.1594) -> (-665.3213, 340.4888)
  circle A302 centre (-667.7025, 353.412) radius 9.8425 construction
  arc A303 (-657.7013, 344.8882) -> (-665.3213, 340.4888) centre (-660.2413, 340.4888) ccw
  line L230 (-655.32, 357.8114) -> (-629.92, 372.4761)
  arc A304 (-622.3, 368.0767) -> (-629.92, 372.4761) centre (-627.38, 368.0767) ccw
  line L231 (-622.3, 368.0767) -> (-622.3, 338.7473)
  arc A305 (-629.92, 334.3479) -> (-622.3, 338.7473) centre (-627.38, 338.7473) ccw
  line L232 (-629.92, 334.3479) -> (-655.32, 349.0126)
  circle A306 centre (-667.7025, 353.412) radius 9.8425 construction
  arc A307 (-655.32, 357.8114) -> (-655.32, 349.0126) centre (-652.78, 353.412) ccw
  line L233 (-665.3212, 366.3353) -> (-665.3212, 395.6647)
  arc A308 (-657.7012, 400.0641) -> (-665.3212, 395.6647) centre (-660.2412, 395.6647) ccw
  line L234 (-657.7012, 400.0641) -> (-632.3012, 385.3994)
  arc A309 (-632.3012, 376.6006) -> (-632.3012, 385.3994) centre (-634.8412, 381) ccw
  line L235 (-632.3012, 376.6006) -> (-657.7012, 361.9359)
  circle A310 centre (-667.7025, 353.412) radius 9.8425 construction
  arc A311 (-665.3212, 366.3353) -> (-657.7012, 361.9359) centre (-660.2412, 366.3353) ccw
  line L236 (-677.7037, 361.9359) -> (-703.1037, 376.6006)
  arc A312 (-703.1037, 385.3994) -> (-703.1037, 376.6006) centre (-700.5637, 381) ccw
  line L237 (-703.1037, 385.3994) -> (-677.7037, 400.0641)
  arc A313 (-670.0837, 395.6647) -> (-677.7037, 400.0641) centre (-675.1637, 395.6647) ccw
  line L238 (-670.0837, 395.6647) -> (-670.0837, 366.3353)
  circle A314 centre (-667.7025, 353.412) radius 9.8425 construction
  arc A315 (-677.7037, 361.9359) -> (-670.0837, 366.3353) centre (-675.1637, 366.3353) ccw
  line L239 (-680.085, 349.0126) -> (-705.485, 334.3479)
  arc A316 (-713.105, 338.7473) -> (-705.485, 334.3479) centre (-708.025, 338.7473) ccw
  line L240 (-713.105, 338.7473) -> (-713.105, 368.0767)
  arc A317 (-705.485, 372.4761) -> (-713.105, 368.0767) centre (-708.025, 368.0767) ccw
  line L241 (-705.485, 372.4761) -> (-680.085, 357.8114)
  circle A318 centre (-667.7025, 353.412) radius 9.8425 construction
  arc A319 (-680.085, 349.0126) -> (-680.085, 357.8114) centre (-682.625, 353.412) ccw
  circle A320 centre (-667.7025, 408.588) radius 9.8425 construction
  line L242 (-680.085, 404.1886) -> (-705.485, 389.5239)
  line L243 (-705.485, 427.6521) -> (-680.085, 412.9874)
  arc A321 (-705.485, 427.6521) -> (-713.105, 423.2527) centre (-708.025, 423.2527) ccw
  line L244 (-713.105, 393.9233) -> (-713.105, 423.2527)
  arc A322 (-713.105, 393.9233) -> (-705.485, 389.5239) centre (-708.025, 393.9233) ccw
  arc A323 (-680.085, 404.1886) -> (-680.085, 412.9874) centre (-682.625, 408.588) ccw
  line L245 (-677.7038, 417.1118) -> (-703.1038, 431.7765)
  line L246 (-670.0838, 450.8406) -> (-670.0838, 421.5112)
  arc A324 (-670.0838, 450.8406) -> (-677.7038, 455.24) centre (-675.1638, 450.8406) ccw
  line L247 (-703.1038, 440.5753) -> (-677.7038, 455.24)
  arc A325 (-703.1038, 440.5753) -> (-703.1038, 431.7765) centre (-700.5638, 436.1759) ccw
  arc A326 (-677.7038, 417.1118) -> (-670.0838, 421.5112) centre (-675.1638, 421.5112) ccw
  line L248 (-665.3213, 421.5112) -> (-665.3213, 450.8406)
  line L249 (-632.3013, 431.7765) -> (-657.7013, 417.1118)
  arc A327 (-632.3013, 431.7765) -> (-632.3013, 440.5753) centre (-634.8413, 436.1759) ccw
  line L250 (-657.7013, 455.24) -> (-632.3013, 440.5753)
  arc A328 (-657.7013, 455.24) -> (-665.3213, 450.8406) centre (-660.2413, 450.8406) ccw
  arc A329 (-665.3213, 421.5112) -> (-657.7013, 417.1118) centre (-660.2413, 421.5112) ccw
  line L251 (-655.32, 412.9874) -> (-629.92, 427.6521)
  line L252 (-629.92, 389.5239) -> (-655.32, 404.1886)
  arc A330 (-629.92, 389.5239) -> (-622.3, 393.9233) centre (-627.38, 393.9233) ccw
  line L253 (-622.3, 423.2527) -> (-622.3, 393.9233)
  arc A331 (-622.3, 423.2527) -> (-629.92, 427.6521) centre (-627.38, 423.2527) ccw
  arc A332 (-655.32, 412.9874) -> (-655.32, 404.1886) centre (-652.78, 408.588) ccw
  line L254 (-657.7012, 400.0641) -> (-632.3012, 385.3994)
  line L255 (-665.3212, 366.3353) -> (-665.3212, 395.6647)
  arc A333 (-665.3212, 366.3353) -> (-657.7012, 361.9359) centre (-660.2412, 366.3353) ccw
  line L256 (-632.3012, 376.6006) -> (-657.7012, 361.9359)
  arc A334 (-632.3012, 376.6006) -> (-632.3012, 385.3994) centre (-634.8412, 381) ccw
  arc A335 (-657.7012, 400.0641) -> (-665.3212, 395.6647) centre (-660.2412, 395.6647) ccw
  circle A336 centre (-667.7025, 463.7639) radius 9.8425 construction
  line L257 (-622.3, 478.4286) -> (-622.3, 449.0992)
  line L258 (-629.92, 444.6998) -> (-655.32, 459.3645)
  arc A337 (-629.92, 444.6998) -> (-622.3, 449.0992) centre (-627.38, 449.0992) ccw
  arc A338 (-655.32, 468.1633) -> (-655.32, 459.3645) centre (-652.78, 463.7639) ccw
  line L259 (-655.32, 468.1633) -> (-629.92, 482.828)
  arc A339 (-622.3, 478.4286) -> (-629.92, 482.828) centre (-627.38, 478.4286) ccw
  line L260 (-657.7012, 510.4159) -> (-632.3012, 495.7513)